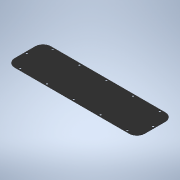
# Autodesk Inventor part: 1XX7_04_00_7(2)_P5
Saved by Autodesk Inventor 2021 (Build 250183000, 183)
## iProperties
Created: 2025-08-26
Part Number: 1XX7_04_00_7(2)_P5
Material: Generic
Catalog Web Link: www.cadenas.de
Description: AE 2.0 Flanschplatte-AE 2.0 Flanschplatte
Vendor: RITTAL
Document SubType Name: Modeling
Designer: psAdmin
Manufacturer: RITTAL
Mass: 117.298 g
Surface Area: 1587.71 cm^2
Volume: 117.298 cm^3
Density: 1 g/cm^3
Appearance: PSOLRGB-176-176-176
Category: PARTsolutions
Company: RITTAL
Title: 1XX7_04_00_7(2)_P5
Author: Cadenas PARTsolutions
Comments: AE 2.0 Flanschplatte
PSOL_IDENT_0: {$CADENAS_DATA/23d-libs/rittal/schaltschranksys/kompakt_schaltschr/parts_ae_2_0/flanschplatte_ae_2_0
PSOL_IDENT_1: .prj},203 {VTYP=3D},{NB=1XX7_04_00_7(2)_P5},{LINA=1XX7_04_00_7(2)_P5},{NN=AE 2.0 Flanschplatte},{DAT
PSOL_IDENT_2: E=28.04.2025 21:11:31},{GEOMDATE=11.04.2025 11:21:47},{VERSION=},{LINEID=180},{WBVAR=DETAIL},{WBNUME
PSOL_IDENT_3: RIC=DETAIL}  {NB=1XX7_04_00_7(2)_P5},{LINA=1XX7_04_00_7(2)_P5},{KT=DUMMY},{BEST=1XX7},{DETAIL=2},{BE
PSOL_IDENT_4: Z1=Neues Kompaktgehäuse},{BEZ2=Stahlblech},{BEZ3=eintürig},{B=440.000},{H=133.000},{T=5},{F=450},{G=
PSOL_IDENT_5: 475},{B1=518.000},{H1=0.000},{T1=210},{F1=450},{G1=475},{S=2.5},{ST=MIN},{GEW=-1.00000001504747e+30}
PSOL_IDENT_6: ,{VERS=7},{CNSECLASS51=27-18-01-02},{CNSECLASS70=27-18-01-01},{CNSECLASS80=27-18-01-01},{CNSETIM40=E
PSOL_IDENT_7: C000261}
NB: 1XX7_04_00_7(2)_P5
NN: AE 2.0 Flanschplatte
NT: AE 2.0 Flanschplatte
NBSYN: $BEST._04_00_$VERS.($DETAIL.)_P5
LINA: 1XX7_04_00_7(2)_P5
CATALOG: Rittal
BEST: 1XX7
DETAIL: niedrig
BEZ1: Neues Kompaktgehäuse
BEZ2: Stahlblech
BEZ3: eintürig
B: 440
H: 133
T: 5
F: 450
G: 475
B1: 518
H1: 0
T1: 210
F1: 450
G1: 475
S: 2.5
ST: 0
GEW: -1.00000001504747e+30
VERS: 7
CNSECLASS70: 27-18-01-01
CNSECLASS80: 27-18-01-01
SUPPLIER: RITTAL
ARTICLENO: 1XX7_04_00_7(2)_P5
BOMINFO: 1XX7_04_00_7(2)_P5
CREATOR: CADENAS GmbH
Autodesk Inventor part; units mm, degrees
sketch "Sketch_7" plane through (0, 0, 0) normal (0, 1, 0) x (1, 0, 0)
  arc A0 (-267, -42.5) -> (-235, -74.5) centre (-235, -42.5) ccw
  line L0 (-235, -74.5) -> (235, -74.5)
  arc A1 (235, -74.5) -> (267, -42.5) centre (235, -42.5) ccw
  line L1 (267, -42.5) -> (267, 42.5)
  arc A2 (267, 42.5) -> (235, 74.5) centre (235, 42.5) ccw
  line L2 (235, 74.5) -> (-235, 74.5)
  arc A3 (-235, 74.5) -> (-267, 42.5) centre (-235, 42.5) ccw
  line L3 (-267, 42.5) -> (-267, -42.5)
  circle A4 centre (259, 0) radius 3.6
  circle A5 centre (220, -66.5) radius 3.6
  circle A6 centre (220, 66.5) radius 3.6
  circle A7 centre (110, -66.5) radius 3.6
  circle A8 centre (110, 66.5) radius 3.6
  circle A9 centre (0, -66.5) radius 3.6
  circle A10 centre (0, 66.5) radius 3.6
  circle A11 centre (-110, -66.5) radius 3.6
  circle A12 centre (-110, 66.5) radius 3.6
  circle A13 centre (-220, -66.5) radius 3.6
  circle A14 centre (-220, 66.5) radius 3.6
  circle A15 centre (-259, 0) radius 3.6
  constraints: 16 centre point, 8 end point, 8 point on circle
extrude "Extrusion1" add sketch "Sketch_7" along normal blind 1.5
ref_plane "FP_XY" through (0, 0, 0) normal (0, -1, 0) x (1, 0, 0)
ref_plane "FP_YZ" through (0, 0, 0) normal (1, 0, 0) x (0, 0, 1)
ref_plane "FP_ZX" through (0, 0, 0) normal (0, 0, 1) x (0, -1, 0)
ref_plane "to_Bolt_1_XY" through (-259, 0, 0) normal (0, 1, 0) x (1, 0, 0)
ref_plane "to_Bolt_1_YZ" through (-259, 0, 0) normal (1, 0, 0) x (0, 0, -1)
ref_plane "to_Bolt_1_ZX" through (-259, 0, 0) normal (0, 0, -1) x (0, 1, 0)
ref_plane "to_Bolt_1_1_XY" through (-220, 0, -66.5) normal (0, 1, 0) x (1, 0, 0)
ref_plane "to_Bolt_1_1_YZ" through (-220, 0, -66.5) normal (1, 0, 0) x (0, 0, -1)
ref_plane "to_Bolt_1_1_ZX" through (-220, 0, -66.5) normal (0, 0, -1) x (0, 1, 0)
ref_plane "to_Bolt_1_10_XY" through (220, 0, 66.5) normal (0, 1, 0) x (1, 0, 0)
ref_plane "to_Bolt_1_10_YZ" through (220, 0, 66.5) normal (1, 0, 0) x (0, 0, -1)
ref_plane "to_Bolt_1_10_ZX" through (220, 0, 66.5) normal (0, 0, -1) x (0, 1, 0)
ref_plane "to_Bolt_1_2_XY" through (-110, 0, -66.5) normal (0, 1, 0) x (1, 0, 0)
ref_plane "to_Bolt_1_2_YZ" through (-110, 0, -66.5) normal (1, 0, 0) x (0, 0, -1)
ref_plane "to_Bolt_1_2_ZX" through (-110, 0, -66.5) normal (0, 0, -1) x (0, 1, 0)
ref_plane "to_Bolt_1_3_XY" through (0, 0, -66.5) normal (0, 1, 0) x (1, 0, 0)
ref_plane "to_Bolt_1_3_YZ" through (0, 0, -66.5) normal (1, 0, 0) x (0, 0, -1)
ref_plane "to_Bolt_1_3_ZX" through (0, 0, -66.5) normal (0, 0, -1) x (0, 1, 0)
ref_plane "to_Bolt_1_4_XY" through (110, 0, -66.5) normal (0, 1, 0) x (1, 0, 0)
ref_plane "to_Bolt_1_4_YZ" through (110, 0, -66.5) normal (1, 0, 0) x (0, 0, -1)
ref_plane "to_Bolt_1_4_ZX" through (110, 0, -66.5) normal (0, 0, -1) x (0, 1, 0)
ref_plane "to_Bolt_1_5_XY" through (220, 0, -66.5) normal (0, 1, 0) x (1, 0, 0)
ref_plane "to_Bolt_1_5_YZ" through (220, 0, -66.5) normal (1, 0, 0) x (0, 0, -1)
ref_plane "to_Bolt_1_5_ZX" through (220, 0, -66.5) normal (0, 0, -1) x (0, 1, 0)
ref_plane "to_Bolt_1_6_XY" through (-220, 0, 66.5) normal (0, 1, 0) x (1, 0, 0)
ref_plane "to_Bolt_1_6_YZ" through (-220, 0, 66.5) normal (1, 0, 0) x (0, 0, -1)
ref_plane "to_Bolt_1_6_ZX" through (-220, 0, 66.5) normal (0, 0, -1) x (0, 1, 0)
ref_plane "to_Bolt_1_7_XY" through (-110, 0, 66.5) normal (0, 1, 0) x (1, 0, 0)
ref_plane "to_Bolt_1_7_YZ" through (-110, 0, 66.5) normal (1, 0, 0) x (0, 0, -1)
ref_plane "to_Bolt_1_7_ZX" through (-110, 0, 66.5) normal (0, 0, -1) x (0, 1, 0)
ref_plane "to_Bolt_1_8_XY" through (0, 0, 66.5) normal (0, 1, 0) x (1, 0, 0)
ref_plane "to_Bolt_1_8_YZ" through (0, 0, 66.5) normal (1, 0, 0) x (0, 0, -1)
ref_plane "to_Bolt_1_8_ZX" through (0, 0, 66.5) normal (0, 0, -1) x (0, 1, 0)
ref_plane "to_Bolt_1_9_XY" through (110, 0, 66.5) normal (0, 1, 0) x (1, 0, 0)
ref_plane "to_Bolt_1_9_YZ" through (110, 0, 66.5) normal (1, 0, 0) x (0, 0, -1)
ref_plane "to_Bolt_1_9_ZX" through (110, 0, 66.5) normal (0, 0, -1) x (0, 1, 0)
ref_plane "to_Bolt_2_XY" through (259, 0, 0) normal (0, 1, 0) x (1, 0, 0)
ref_plane "to_Bolt_2_YZ" through (259, 0, 0) normal (1, 0, 0) x (0, 0, -1)
ref_plane "to_Bolt_2_ZX" through (259, 0, 0) normal (0, 0, -1) x (0, 1, 0)
body "Solid1"
